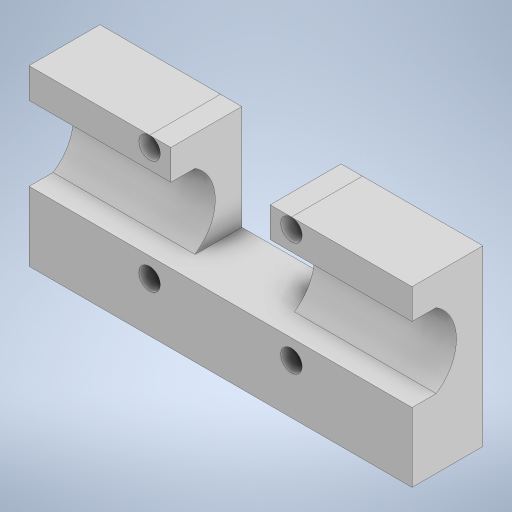
# Autodesk Inventor part: Držák motoru (spodní díl)
Saved by Autodesk Inventor 2024 (Build 280153000, 153)
## iProperties
Created: 2023-08-14
Part Number: Držák motoru (spodní díl)
Material: Všeobecné
Document SubType Name: Modeling
Designer: jaryj
Density: 1 g/cm^3
Appearance: Výchozí
Author: jaryj
Autodesk Inventor part; units mm, degrees
ref_plane "YZ Plane" through (0, 0, 0) normal (1, 0, 0) x (0, 1, 0)
ref_plane "XZ Plane" through (0, 0, 0) normal (0, 1, 0) x (-1, 0, 0)
ref_plane "XY Plane" through (0, 0, 0) normal (0, 0, 1) x (1, 0, 0)
sketch "Náčrt1" plane through (0, 0, 0) normal (0, 0, 1) x (1, 0, 0)
  line L0 (0, 15) -> (-27, 15)
  line L1 (-27, 15) -> (-27, -15)
  line L2 (-27, -15) -> (0, -15)
  line L3 (0, -15) -> (0, 15)
  circle A0 centre (-10, 8) radius 1.5
  line L4 (-14.1616, 0) -> (12.8881, 0)
  circle A1 centre (-10, -8) radius 1.5
  point P0 (0, 0)
  point P1 (0, 0)
  dimension "d13" = 30
  dimension "d14" = 27
  dimension "d15" = 3
  dimension "d18" = 16
  dimension "d23" = 10
  constraints: 10 end point, 2 centre point, 2 horizontal, 2 parallel, 1 coincident, 1 horizontal alignment, 1 midpoint, 1 perpendicular, 1 symmetric about line, 1 vertical, 1 vertical alignment, 2 other
  measures "d13" distance of L0.end L1.end
  measures "d14" distance of L0.start L0.end
  measures "d15" diameter of A0
  measures "d18" distance of A0.centre A1.centre
  measures "d23" distance from line of L3 A0.centre
extrude "Vysunutí2" add sketch "Náčrt1" along normal blind 10
sketch "Náčrt2" plane through (-27, -15, 0) normal (-1, 0, 0) x (0, 0, 1)
  line L0 (10, 0) -> (10, 30) projected
  line L1 (10, 20) -> (6.6834, 20)
  line L2 (10, 10) -> (6.6834, 10)
  arc A0 (6.6834, 20) -> (6.6834, 10) centre (10, 15) ccw
  line L3 (0, 30) -> (0, 0) projected
  line L4 (10, 9.75) -> (6.6088, 9.75)
  arc A1 (6.6088, 20.25) -> (6.6088, 9.75) centre (10, 15) ccw
  line L5 (6.6088, 20.25) -> (10, 20.25)
  point P0 (0, 15)
  point P1 (0, 15)
  dimension "d26" = 10
  dimension "d27" = 6
  dimension "d28" = 0.25
  constraints: 8 end point, 4 point on circle, 2 centre point, 2 point on line, 2 vertical alignment, 1 horizontal, 1 horizontal alignment, 1 midpoint, 1 perpendicular, 2 other
  measures "d26" distance between parallel lines of L2 L1
  measures "d27" radius of A0
  measures "d28" radial gap between concentric circles of A0 A1
extrude "Vysunutí3" cut sketch "Náčrt2" against normal through all
sketch "Náčrt3" plane through (0, 0, 10) normal (0, 0, 1) x (1, 0, 0)
  line L0 (0, 15) -> (-27, 15) projected
  circle A0 centre (-10, 8) radius 1.5 projected
  line L1 (0, -5.25) -> (-27, -5.25) projected
  line L2 (0, 5.25) -> (0, 15) projected
  line L3 (-7, -5.25) -> (-7, 9.5)
  line L4 (-7, 9.5) -> (-27, 9.5)
  line L5 (-27, 15) -> (-27, 5.25) projected
  line L6 (0, 5.25) -> (0, -5.25) projected
  point P0 (0, 0)
  dimension "d34" = 3
  constraints: 4 end point, 1 perpendicular, 1 point on line, 1 tangent, 1 vertical, 1 vertical alignment
  measures "d34" distance from line of L3 A0.centre
extrude "Vysunutí4" cut sketch "Náčrt3" against normal through all contours L2 L6 L1 L3 L4 L5 L0
mirror "Zrcadlit1" about plane through (0, -15, 0) normal (1, 0, 0)
